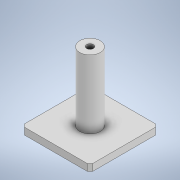
# Autodesk Inventor part: Leg
Saved by Autodesk Inventor 2020.3 (Build 243373010, 373A)
## iProperties
Created: 2020-10-30
Part Number: Leg
Material: Generic
Document SubType Name: Modeling
Designer: Naude Conradie
Density: 1 g/cm^3
Appearance: Default
Author: Naude Conradie
Autodesk Inventor part; units mm, degrees
ref_plane "YZ Plane" through (0, 0, 0) normal (1, 0, 0) x (0, 1, 0)
ref_plane "XZ Plane" through (0, 0, 0) normal (0, 1, 0) x (-1, 0, 0)
ref_plane "XY Plane" through (0, 0, 0) normal (0, 0, 1) x (1, 0, 0)
sketch "Sketch1" plane through (0, 0, 0) normal (0, 1, 0) x (-1, 0, 0)
  circle A0 centre (0, 0) radius 7.5
  dimension "d0" = 15
  constraints: 1 centre point, 1 coincident
  measures "d0" diameter of A0
extrude "Extrusion1" add sketch "Sketch1" along normal blind 50
sketch "Sketch2" plane through (0, 0, 0) normal (0, -1, 0) x (1, 0, 0)
  line L0 (-25, 25) -> (25, 25)
  line L1 (25, 25) -> (25, -25)
  line L2 (25, -25) -> (-25, -25)
  line L3 (-25, -25) -> (-25, 25)
  point P0 (0, 0)
  dimension "d3" = 50
  dimension "d4" = 50
  dimension "d5" = 25
  dimension "d6" = 25
  constraints: 8 end point, 2 parallel, 1 horizontal, 1 perpendicular
  measures "d3" distance of L0.end L1.end
  measures "d4" distance of L0.start L0.end
  measures "d5" distance from line of L0 point (0, 0)
  measures "d6" distance from line of L3 point (0, 0)
extrude "Extrusion2" add sketch "Sketch2" along normal blind 5
chamfer "Chamfer1" distance 2 angle 45 4 edges at (25, -2.5, 25) (-25, -2.5, 25) (-25, -2.5, -25) (25, -2.5, -25)
sketch "Sketch3" plane through (0, 50, 0) normal (0, 1, 0) x (1, 0, 0)
  point P0 (0, 0)
  point P1 (0, 0)
  constraints: 1 coincident
hole "Hole1" at (0, 50, 0) direction (0, -1, 0) diameter 5 depth 10 tip angle 118
body "Solid1"
